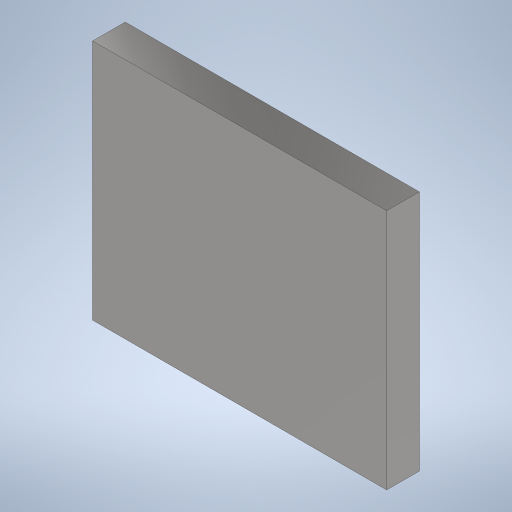
# Autodesk Inventor part: Gegenstück_Magnet
Saved by Autodesk Inventor 2024 (Build 280153000, 153)
## iProperties
Created: 2025-04-08
Part Number: Gegenstück_Magnet
Material: Eisen, schmiedbar
Document SubType Name: Modeling
Designer: fynnb
Density: 7.15 g/cm^3
Appearance: Halbpoliert
Author: fynnb
Autodesk Inventor part; units mm, degrees
ref_plane "YZ Plane" through (0, 0, 0) normal (1, 0, 0) x (0, 1, 0)
ref_plane "XZ Plane" through (0, 0, 0) normal (0, 1, 0) x (-1, 0, 0)
ref_plane "XY Plane" through (0, 0, 0) normal (0, 0, 1) x (1, 0, 0)
sketch "Skizze1" plane through (0, 0, 0) normal (0, 1, 0) x (-1, 0, 0)
  line L0 (8.4971, 66.5651) -> (-81.5029, 66.5651)
  line L1 (-81.5029, 66.5651) -> (-81.5029, -7.4349)
  line L2 (-81.5029, -7.4349) -> (8.4971, -7.4349)
  line L3 (8.4971, -7.4349) -> (8.4971, 66.5651)
  point P0 (0, 0)
  dimension "d0" = 74
  dimension "d1" = 90
  constraints: 8 end point, 2 parallel, 1 horizontal, 1 perpendicular
  measures "d0" distance of L2.end L0.start
  measures "d1" distance of L1.end L2.end
extrude "Extrusion1" add sketch "Skizze1" along normal blind 10
